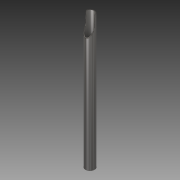
# Autodesk Inventor part: pin
Saved by Autodesk Inventor 2017.3 (Build 213256000, 256)
## iProperties
Part Number: pin
Material: Generisch
Document SubType Name: Modeling
Designer: Ljubko
Density: 1 g/cm^3
Appearance: Vorgabe
Author: Ljubko
Autodesk Inventor part; units mm, degrees
ref_plane "YZ Plane" through (0, 0, 0) normal (1, 0, 0) x (0, 1, 0)
ref_plane "XZ Plane" through (0, 0, 0) normal (0, 1, 0) x (-1, 0, 0)
ref_plane "XY Plane" through (0, 0, 0) normal (0, 0, 1) x (1, 0, 0)
sketch "Skizze1" plane through (0, 0, 0) normal (0, 0, 1) x (1, 0, 0)
  arc A0 (0.0104, -0.4999) -> (-0.0104, -0.4999) centre (0, 0) ccw
  arc A1 (0.0104, -0.4499) -> (-0.0104, -0.4499) centre (0, 0) ccw
  line L0 (-0.0104, -0.4499) -> (-0.0104, -0.4999)
  line L1 (0.0104, -0.4499) -> (0.0104, -0.4999)
  point P0 (-0.0054, 0)
  point P1 (0.0054, 0)
  dimension "d0" = 1
  dimension "d1" = 0.9
  dimension "d18" = 0.0209
  constraints: 4 end point, 4 point on circle, 2 centre point, 1 parallel
  measures "d0" diameter of A0
  measures "d1" diameter of A1
  measures "d18" distance between parallel lines of L1 L0
extrude "Extrusion1" add sketch "Skizze1" along normal blind 14.8
sketch "Skizze2" plane through (0, 0, 0) normal (1, 0, 0) x (0, 1, 0)
  line L0 (-0.5, 0) -> (-0.5, 14.8)
  line L1 (-0.5, 12.6) -> (-0.0804, 13.3267)
  line L2 (0, 13.9708) -> (0, 13.6267)
  line L3 (0, 13.9708) -> (0.0666, 14.8632)
  arc A0 (-0.0804, 13.3267) -> (0, 13.6267) centre (-0.6, 13.6267) ccw
  line L4 (0.45, 0) -> (0.45, 14.8) projected
  line L5 (0.45, 14.8) -> (0.5, 14.8) projected
  line L6 (0.5, 14.8) -> (0.5, 0) projected
  line L7 (0.5, 0) -> (0.45, 0) projected
  arc A1 (0.0666, 14.8632) -> (-0.5, 12.6) centre (-0.4472, 13.7893) ccw
  point P0 (0, 0)
  point P1 (0, 13.466)
  dimension "d8" = 30
  dimension "d10" = 0.6
  constraints: 8 end point, 4 point on circle, 2 centre point, 2 point on line, 2 tangent
  measures "d8" angle of L0 L1
  measures "d10" radius of A0
extrude "Extrusion3" cut sketch "Skizze2" along normal through all both and the other way through all contours A1 L3 L2 A0 L1
